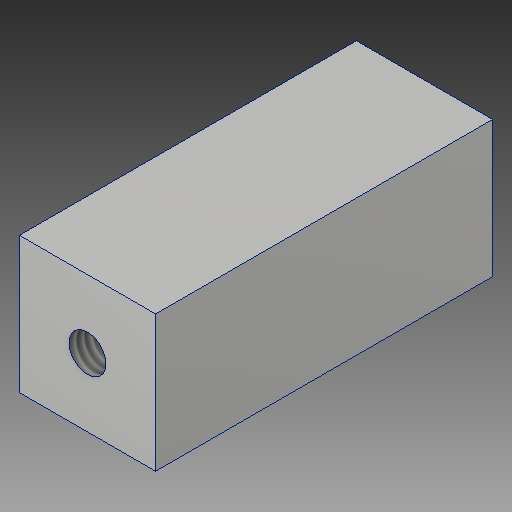
# Autodesk Inventor part: espassador_soprador
Saved by Autodesk Inventor 2018 (Build 220112000, 112)
## iProperties
Created: 2018-05-10
Part Number: espassador_soprador
Material: Alumínio 6061
Document SubType Name: Modeling
Designer: Georgines
Density: 2.7 g/cm^3
Appearance: Alumínio - Plano
Author: Georgines
Autodesk Inventor part; units mm, degrees
ref_plane "YZ Plane" through (0, 0, 0) normal (1, 0, 0) x (0, 1, 0)
ref_plane "XZ Plane" through (0, 0, 0) normal (0, 1, 0) x (-1, 0, 0)
ref_plane "XY Plane" through (0, 0, 0) normal (0, 0, 1) x (1, 0, 0)
sketch "Esboço1" plane through (0, 0, 0) normal (0, 0, 1) x (1, 0, 0)
  line L0 (4.9347, -7.2977) -> (-6.5153, -7.2977) projected
  line L1 (4.9347, -7.2977) -> (4.9347, 10.1323) projected
  line L2 (4.9347, 10.1323) -> (2.5947, 10.1323) projected
  line L3 (2.5947, 10.1323) -> (-0.1453, 0.6423) projected
  line L4 (-0.1453, 0.6423) -> (-0.1453, -1.2977) projected
  arc A0 (-2.7953, -1.2977) -> (-0.1453, -1.2977) centre (-1.4703, -1.2977) ccw projected
  line L5 (-2.7953, -1.2977) -> (-2.7953, 2.6323) projected
  line L6 (-2.7953, 2.6323) -> (-6.5153, 2.6323) projected
  line L7 (-6.5153, 2.6323) -> (-6.5153, -7.2977) projected
  line L8 (-7.4703, 4.7023) -> (4.5297, 4.7023)
  line L9 (4.5297, 4.7023) -> (4.5297, -7.2977)
  line L10 (4.5297, -7.2977) -> (-7.4703, -7.2977)
  line L11 (-7.4703, -7.2977) -> (-7.4703, 4.7023)
  line L12 (-7.4703, 4.7023) -> (4.5297, -7.2977) construction
  line L13 (4.5297, 4.7023) -> (-7.4703, -7.2977) construction
  point P0 (0, 0)
  dimension "d0" = 12
  dimension "d1" = 12
  constraints: 12 end point, 2 midpoint, 2 parallel, 1 horizontal, 1 perpendicular
  measures "d0" distance of L9.end L10.end
  measures "d1" distance of L8.end L9.end
ref_plane "Plano de trabalho1" through (-14.4853, -144.1477, 29.69) normal (0, 0, -1) x (0, 1, 0)
extrude "Extrusão1" add sketch "Esboço1" along normal up to surface (29.69 mm away) contours L0 L7 L6 L5 A0 L4 L3 L8 L9 | L10 L11 L8 L3 L4 A0 L5 L6 L7
sketch "Esboço3" plane through (0, 0, 0) normal (0, 0, -1) x (-1, 0, 0)
  line L0 (-4.5297, 4.7023) -> (7.4703, 4.7023) projected
  line L1 (7.4703, -7.2977) -> (-4.5297, -7.2977) projected
  line L2 (-4.5297, -7.2977) -> (-4.5297, 4.7023) construction
  line L3 (-4.5297, 4.7023) -> (7.4703, -7.2977) construction
  line L4 (7.4703, 4.7023) -> (-4.5297, -7.2977) construction
  circle A0 centre (1.4703, -1.2977) radius 3 construction
  dimension "d13" = 6
  constraints: 4 end point, 1 centre point, 1 midpoint, 1 perpendicular
  measures "d13" diameter of A0
hole "Furo2" at (-1.4703, -1.2977, 0) direction (0, 0, 1) diameter 3.242 depth 12 tip angle 118 thread size "M4x0.7" class "6H" standard "ISO Metric profile"
sketch "Esboço5" plane through (-7.4703, 4.7023, 29.69) normal (0, 0, 1) x (1, 0, 0)
  circle A0 centre (6, -6) radius 1.621 projected
  circle A1 centre (6, -6) radius 3.7537 construction
  constraints: 1 centre point, 1 coincident
hole "Furo3" at (-1.4703, -1.2977, 29.69) direction (0, 0, -1) diameter 3.242 depth 12 tip angle 118 thread size "M4x0.7" class "6H" standard "ISO Metric profile"
